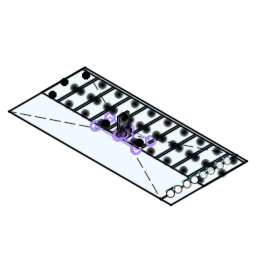
RIS-fusion360 (Autodesk Fusion 360 design; units mm, degrees)
Autodesk Fusion 360 part; units mm, degrees
sketch "Sketch1" plane through (0, 0, 0) normal (1, 0, 0) x (0, 1, 0)
  line L0 (9.4, 3.95) -> (-9.4, 3.95)
  line L1 (-9.4, 3.95) -> (-9.4, -3.95)
  line L2 (-9.4, -3.95) -> (9.4, -3.95)
  line L3 (9.4, -3.95) -> (9.4, 3.95)
  line L4 (9.4, 3.95) -> (-9.4, -3.95) construction
  line L5 (-9.4, 3.95) -> (9.4, -3.95) construction
  circle A0 centre (0, -0.1) radius 1.45
  line L6 (0, 3.95) -> (0, -3.95) construction
  line L7 (0, -3.95) -> (0, -7.55) construction
  line L8 (0, -7.55) -> (-2.05, -7.55)
  line L9 (0, -7.55) -> (2.05, -7.55)
  line L10 (-2.05, -7.55) -> (-2.05, -3.95)
  line L11 (2.05, -7.55) -> (2.05, -3.95)
  line L12 (0, -7.55) -> (-7.5, -7.55)
  line L13 (0, -7.55) -> (7.5, -7.55)
  line L14 (-7.5, -7.55) -> (-7.5, -10)
  line L15 (-7.5, -10) -> (7.5, -10)
  line L16 (7.5, -10) -> (7.5, -7.55)
  circle A1 centre (0, 3.3786) radius 5.7286
  point P0 (0, -3.95)
  point P1 (0, -2.35)
  point P2 (5.7, 3.95)
  point P3 (-5.7, 3.95)
  dimension "d1" = 18.8
  dimension "d2" = 7.9
  dimension "d3" = 2.9
  dimension "d4" = 4.05
  dimension "d7" = 3.6
  dimension "d8" = 2.05
  dimension "d9" = 2.05
  dimension "d10" = 7.5
  dimension "d11" = 7.5
  dimension "d12" = 2.45
  dimension "d19" = 6.3
  dimension "d20" = 5.7
  dimension "d21" = 5.7
  constraint horizontal L0
  constraint perpendicular L0 L1
  constraint parallel L0 L2
  constraint parallel L1 L3
  constraint coincident L4 origin
  constraint coincident L5 origin
  constraint midpoint L0 L6.start
  constraint coincident A0.centre L6
  constraint coincident P0 L6.end
  constraint midpoint L2 P0
  constraint perpendicular L2 L7
  constraint perpendicular L7 L8
  constraint perpendicular L7 L9
  constraint coincident L2 L10.end
  constraint perpendicular L2 L10
  constraint coincident L2 L11.end
  constraint perpendicular L2 L11
  constraint perpendicular L7 L12
  constraint perpendicular L7 L13
  constraint perpendicular L12 L14
  constraint perpendicular L14 L15
  constraint vertical L16
  constraint coincident L6 P1
  constraint coincident L0 P2
  constraint coincident L0 P3
  constraint coincident P2 A1
  constraint coincident P1 A1
  constraint coincident P3 A1
  measures "d1" distance of L0.start L0.end
  measures "d2" distance of L0.start L2.end
  measures "d3" diameter of A0
  measures "d4" distance of L0 A0.centre
  measures "d7" distance of P0 L7.end
  measures "d8" distance of L7.end L8.end
  measures "d9" distance of L7.end L9.end
  measures "d10" distance of L7.end L12.end
  measures "d11" distance of L7.end L13.end
  measures "d12" distance of L13.end L15.end
  measures "d19" distance of L0 P1
  measures "d20" distance of L6.start P2
  measures "d21" distance of L6.start P3
extrude "Extrude1" add sketch "Sketch1" along normal blind 4.5 contours A0 makes body 1
extrude "Extrude2" add sketch "Sketch1" against normal blind 2.5 separate body contours L0 L1 L2 L3 A1 | L2 L8 L9 L10 L11 L12 L13 makes body 2
extrude "Extrude4" add sketch "Sketch1" against normal blind 1.2 contours L0 A1 picked at (0.0361, 3.082) bodies 2 1
extrude "Extrude3" add sketch "Sketch1" against normal blind 7 contours L8 L9 L12 L13 L14 L15 L16 bodies 2
sketch "Sketch2" plane through (0, 0, 0) normal (1, 0, 0) x (0, 1, 0)
  circle A0 centre (0, -0.1) radius 1.45
  line L0 (-9.4, 3.95) -> (-9.4, -3.95)
  line L1 (-9.4, -3.95) -> (-2.05, -3.95)
  line L2 (-2.05, -3.95) -> (-2.05, -7.55)
  line L3 (-2.05, -7.55) -> (-7.5, -7.55)
  line L4 (-7.5, -7.55) -> (-7.5, -10)
  line L5 (-7.5, -10) -> (7.5, -10)
  line L6 (7.5, -10) -> (7.5, -7.55)
  line L7 (7.5, -7.55) -> (2.05, -7.55)
  line L8 (2.05, -7.55) -> (2.05, -3.95)
  line L9 (2.05, -3.95) -> (9.4, -3.95)
  line L10 (9.4, -3.95) -> (9.4, 3.95)
  line L11 (9.4, 3.95) -> (-9.4, 3.95)
  line L12 (-7.5, -8.775) -> (7.5, -8.775)
  circle A1 centre (0, -0.1) radius 1.65
  line L13 (9.6, -3.95) -> (9.6, 4.15)
  line L14 (9.6, 4.15) -> (-9.6, 4.15)
  line L15 (-9.6, 4.15) -> (-9.6, -3.95)
  line L16 (-2.05, -7.35) -> (-7.5, -7.35)
  line L17 (7.5, -7.35) -> (2.05, -7.35)
  line L18 (-9.6, -4.15) -> (-7.5, -7.35)
  line L19 (9.6, -4.15) -> (7.5, -7.35)
  line L20 (-9.4, -4.15) -> (-2.25, -4.15)
  line L21 (-2.25, -4.15) -> (-2.25, -7.55)
  line L22 (2.25, -7.55) -> (2.25, -4.15)
  line L23 (2.25, -4.15) -> (9.4, -4.15)
  line L24 (-9.4, -4.15) -> (-9.6, -4.15)
  line L25 (9.4, -4.15) -> (9.6, -4.15)
  line L26 (-2.05, -7.35) -> (2.05, -7.35)
  line L27 (-9.6, -3.95) -> (-19.4, -3.95)
  line L28 (-19.4, -3.95) -> (-19.4, 8.95)
  line L29 (-19.4, 8.95) -> (19.4, 8.95)
  line L30 (9.6, -3.95) -> (19.4, -3.95)
  line L31 (19.4, -3.95) -> (19.4, 8.95)
  line L32 (19.4, -3.95) -> (7.5, -7.35)
  line L33 (-19.4, -3.95) -> (-7.5, -7.35)
  line L34 (9.6, -3.95) -> (9.6, -4.15)
  line L35 (-9.6, -3.95) -> (-9.6, -4.15)
  circle A2 centre (-14.4, 1.85) radius 2.1
  line L36 (-9.4, 1.85) -> (-19.4, 1.85) construction
  line L37 (0, 3.95) -> (0, 8.95) construction
  circle A3 centre (14.4, 1.85) radius 2.1
  line L38 (-2.05, -3.95) -> (-9.4, -3.95)
  dimension "d29" = 0.2
  dimension "d45" = 0.2
  dimension "d46" = 0.2
  dimension "d47" = 0.2
  dimension "d48" = 0.2
  dimension "d49" = 0.2
  dimension "d60" = 5
  dimension "d63" = 10
  dimension "d68" = 4.2
  dimension "d99" = 5.8
  constraint midpoint L4 L12.start
  constraint midpoint L6 L12.end
  constraint parallel L20 L24
  constraint parallel L23 L25
  constraint perpendicular L8 L26
  constraint perpendicular L15 L27
  constraint perpendicular L27 L28
  constraint perpendicular L28 L29
  constraint perpendicular L13 L30
  constraint perpendicular L30 L31
  constraint equal L27 L30
  constraint perpendicular L30 L34
  constraint perpendicular L27 L35
  constraint coincident L28 L36.end
  constraint perpendicular L28 L36
  constraint midpoint A2.centre L36
  constraint midpoint L11 L37.start
  constraint midpoint L29 L37.end
  constraint symmetric A2 L37 A3
  constraint coincident L0 L36.start
  measures "d60" distance of L11 L29
  measures "d63" distance of L0 L28
  measures "d68" diameter of A2
  measures "d99" distance of L36 L38
extrude "Extrude5" add sketch "Sketch2" along normal blind 8 separate body contours L0 L1 L2 L8 L9 L10 L11 L26 L38 | L0 L1 L2 L8 L9 L10 L11 L13 L14 L15 L16 L17 L20 L21 L22 L23 L24 L25 L34 L35 L38 | L16 L18 L20 L21 L24 | L18 L27 L33 L35 | L17 L19 L22 L23 L25 | L13 L14 L15 L27 L28 L29 L30 L31 | L19 L30 L32 L34 makes body 3
sketch "Sketch3" plane through (-2.5, 0, 0) normal (-1, 0, 0) x (0, -1, 0)
  line L0 (9.4, -3.95) -> (9.4, 3.95)
  line L1 (9.4, 3.95) -> (5.7, 3.95)
  arc A0 (-5.7, 3.95) -> (5.7, 3.95) centre (0, 3.3786) ccw
  line L2 (-5.7, 3.95) -> (-9.4, 3.95)
  line L3 (-9.4, 3.95) -> (-9.4, -3.95)
  line L4 (-9.4, -3.95) -> (-2.05, -3.95)
  line L5 (-2.05, -3.95) -> (-2.05, -7.55)
  line L6 (-2.05, -7.55) -> (2.05, -7.55)
  line L7 (2.05, -7.55) -> (2.05, -3.95)
  line L8 (2.05, -3.95) -> (9.4, -3.95)
  arc A1 (-5.7, 3.95) -> (5.7, 3.95) centre (0, 3.3786) ccw
  line L9 (5.7, 3.95) -> (-5.7, 3.95)
  arc A2 (-5.501, 3.93) -> (5.501, 3.93) centre (0, 3.3786) ccw
  line L10 (-5.501, 3.93) -> (5.501, 3.93)
  line L11 (-2.05, -3.95) -> (2.05, -3.95)
  line L12 (-9.4, -3.95) -> (-2.05, -3.95) construction
  line L13 (-2.05, -3.95) -> (-2.05, -7.55) construction
  line L14 (2.05, -7.55) -> (2.05, -3.95) construction
  line L15 (2.05, -3.95) -> (9.4, -3.95) construction
  line L16 (-9.4, 3.95) -> (-9.4, -3.95) construction
  line L17 (9.4, -3.95) -> (9.4, 3.95) construction
  line L18 (7.5, -7.55) -> (2.05, -7.55)
  line L19 (2.05, -7.55) -> (-2.05, -7.55)
  line L20 (-2.05, -7.55) -> (-7.5, -7.55)
  line L21 (-7.55, -7.35) -> (-2.05, -7.35)
  line L22 (7.55, -7.35) -> (2.05, -7.35)
  line L23 (19.4, -3.95) -> (19.4, 8.95)
  line L24 (19.4, 8.95) -> (-19.4, 8.95)
  line L25 (-19.4, 8.95) -> (-19.4, -3.95)
  line L26 (-19.4, -3.95) -> (-7.55, -7.35)
  line L27 (19.4, -3.95) -> (7.55, -7.35)
  line L28 (-9.4, -3.95) -> (-19.4, -3.95) construction
  line L29 (9.4, -3.95) -> (19.4, -3.95) construction
  dimension "d34" = 0.2
  dimension "d35" = 0.2
  dimension "d56" = 5.5
  dimension "d57" = 10
  dimension "d58" = 5.5
  dimension "d62" = 5
  constraint parallel L9 L10
  constraint coincident L4.end L5.start
  constraint coincident L7.end L8.start
  constraint coincident L13 L21.end
  constraint perpendicular L13 L21
  constraint coincident L14 L22.end
  constraint perpendicular L14 L22
  constraint perpendicular L23 L24
  constraint coincident L3.end L4.start
  constraint perpendicular L25 L28
  constraint coincident L0.start L8.end
  constraint perpendicular L23 L29
  constraint horizontal L24
  constraint vertical L25
  constraint equal L28 L29
  measures "d34" distance of L20 L21
  measures "d35" distance of L18 L22
  measures "d56" distance of L21.start L21.end
  measures "d57" distance of L23.start L0.start
  measures "d58" distance of L22.start L22.end
  measures "d62" distance of L9 L24
extrude "Extrude6" add sketch "Sketch3" against normal up to surface (1.1 mm away) separate body contours A2 L10 makes body 4
extrude "Extrude7" add sketch "Sketch3" along normal blind 3 separate body contours L0 L1 A0 L2 L3 L4 L8 A1 L11 | L0 L1 L2 L3 L4 L5 L7 L8 L9 L21 L22 L23 L24 L25 L26 L27 | A0 A1 L9 | A2 L10 makes body 5
combine "Combine1" operation add target body 4 tool bodies 5
extrude "Extrude10" add sketch "Sketch2" against normal up to surface (2.3 mm away) contours L16 L18 L20 L21 L24 | L18 L27 L33 L35 | L17 L19 L22 L23 L25 | L13 L14 L15 L27 L28 L29 L30 L31 | L19 L30 L32 L34 | A2 | A3 bodies 3
extrude "Extrude15" cut 2 faces at (0, 13.5612, 2.607) (0, -13.9454, 2.4562) along direction (1, 0, 0) up to surface end surface through (-2.3, 0, 0) normal (-1, 0, 0) offset 0 on bodies 3 bodies 3
sketch "Sketch5" plane through (0, 0, 8.95) normal (0, 0, 1) x (-1, 0, 0)
  line L0 (2.3, 19.4) -> (-8, 19.4)
  line L1 (-8, 19.4) -> (-8, -19.4)
  line L2 (-8, -19.4) -> (2.3, -19.4)
  line L3 (2.3, -19.4) -> (2.3, 19.4)
  line L4 (-4.6, -19.4) -> (-4.6, 19.4)
  dimension "d94" = 3.4
  constraint coincident L2 L4.start
  constraint coincident L0 L4.end
  constraint perpendicular L0 L4
  measures "d94" distance of L1 L4
extrude "Extrude9" add sketch "Sketch5" along normal blind 58 separate body contours L0 L2 L3 L4 makes body 6
sketch "Sketch7" plane through (-5.5, 0, 0) normal (-1, 0, 0) x (0, -1, 0)
  line L0 (19.4, 8.95) -> (-19.4, 8.95)
  line L1 (-19.4, 8.95) -> (-19.4, -3.95)
  line L2 (-19.4, -3.95) -> (-7.55, -7.35)
  line L3 (-7.55, -7.35) -> (-2.05, -7.35)
  line L4 (-2.05, -7.35) -> (-2.05, -3.95)
  line L5 (-2.05, -3.95) -> (2.05, -3.95)
  line L6 (2.05, -3.95) -> (2.05, -7.35)
  line L7 (2.05, -7.35) -> (7.55, -7.35)
  line L8 (7.55, -7.35) -> (19.4, -3.95)
  line L9 (19.4, -3.95) -> (19.4, 8.95)
  circle A0 centre (14.4, 1.85) radius 2.1
  circle A1 centre (-14.4, 1.85) radius 2.1
extrude "Extrude11" cut sketch "Sketch7" against normal up to surface (3 mm away) contours A0 | A1 bodies 4
sketch "Sketch8" plane through (4.6, 0, 0) normal (1, 0, 0) x (0, 1, 0)
  line L0 (-19.4, 8.95) -> (19.4, 8.95)
  line L1 (19.4, 8.95) -> (19.4, 66.95)
  line L2 (19.4, 66.95) -> (-19.4, 66.95)
  line L3 (-19.4, 66.95) -> (-19.4, 8.95)
  line L4 (0, 66.95) -> (0, 8.95) construction
  circle A0 centre (-13, 23.95) radius 2.25
  circle A1 centre (13, 23.95) radius 2.25
  circle A2 centre (0, 58.95) radius 2.25
  line L5 (19.4, 8.95) -> (-19.4, 8.95)
  dimension "d95" = 4.5
  dimension "d100" = 13
  dimension "d101" = 15
  dimension "d102" = 4.5
  dimension "d103" = 50
  constraint midpoint L2 L4.start
  constraint midpoint L0 L4.end
  constraint symmetric L4 A0 A1
  constraint coincident L4 A2.centre
  measures "d95" diameter of A0
  measures "d100" distance of L4 A0.centre
  measures "d101" distance of L0 A0.centre
  measures "d102" diameter of A2
  measures "d103" distance of A2.centre L5
extrude "Extrude16" cut sketch "Sketch8" against normal up to surface (6.9 mm away) contours A0 | A1 | A2 bodies 6
combine "Combine4" operation add target body 3 tool bodies 6
sketch "Motor Mount" plane through (0, 0, 0) normal (0, 0, 1) x (1, 0, 0)
  line L0 (80, 29) -> (-80, 29)
  line L1 (-80, 29) -> (-80, -29)
  line L2 (-80, -29) -> (80, -29)
  line L3 (80, -29) -> (80, 29)
  circle A0 centre (0, -20) radius 2.15
  circle A1 centre (-67, 0) radius 2.15
  line L4 (-47, 0) -> (-47, -7.6)
  line L5 (-47, -7.6) -> (-36.1, -7.6)
  line L6 (-36.1, -7.6) -> (-36.1, -5.5)
  line L7 (-36.1, -5.5) -> (-28.1, -5.5)
  line L8 (-28.1, -5.5) -> (-28.1, -7.6)
  line L9 (-28.1, -7.6) -> (0, -7.6)
  line L10 (0, 0) -> (0, -29) construction
  line L11 (0, 0) -> (-80, 0) construction
  line L12 (0, 1.75) -> (0, 22.5) construction
  line L13 (47, 0) -> (47, -7.6)
  line L14 (47, -7.6) -> (36.1, -7.6)
  line L15 (36.1, -7.6) -> (36.1, -5.5)
  line L16 (36.1, -5.5) -> (28.1, -5.5)
  line L17 (28.1, -5.5) -> (28.1, -7.6)
  line L18 (28.1, -7.6) -> (0, -7.6)
  line L19 (1.75, 0) -> (22.5, 0) construction
  line L20 (-47, 0) -> (-47, 7.6)
  line L21 (-47, 7.6) -> (-36.1, 7.6)
  line L22 (-36.1, 7.6) -> (-36.1, 5.5)
  line L23 (-36.1, 5.5) -> (-28.1, 5.5)
  line L24 (-28.1, 5.5) -> (-28.1, 7.6)
  line L25 (-28.1, 7.6) -> (0, 7.6)
  line L26 (47, 0) -> (47, 7.6)
  line L27 (47, 7.6) -> (36.1, 7.6)
  line L28 (36.1, 7.6) -> (36.1, 5.5)
  line L29 (36.1, 5.5) -> (28.1, 5.5)
  line L30 (28.1, 5.5) -> (28.1, 7.6)
  line L31 (28.1, 7.6) -> (0, 7.6)
  circle A2 centre (65, 0) radius 2.15
  circle A3 centre (0, 20) radius 2.15
  line L32 (-28.35, 7.85) -> (0, 7.85)
  line L33 (28.35, 7.85) -> (0, 7.85)
  line L34 (28.35, 5.75) -> (28.35, 7.85)
  line L35 (35.85, 5.75) -> (28.35, 5.75)
  line L36 (35.85, 7.85) -> (35.85, 5.75)
  line L37 (47.25, 7.85) -> (35.85, 7.85)
  line L38 (47.25, 0) -> (47.25, 7.85)
  line L39 (47.25, 0) -> (47.25, -7.85)
  line L40 (47.25, -7.85) -> (35.85, -7.85)
  line L41 (35.85, -7.85) -> (35.85, -5.75)
  line L42 (35.85, -5.75) -> (28.35, -5.75)
  line L43 (28.35, -5.75) -> (28.35, -7.85)
  line L44 (28.35, -7.85) -> (0, -7.85)
  line L45 (-28.35, -7.85) -> (0, -7.85)
  line L46 (-28.35, -5.75) -> (-28.35, -7.85)
  line L47 (-35.85, -5.75) -> (-28.35, -5.75)
  line L48 (-35.85, -7.85) -> (-35.85, -5.75)
  line L49 (-47.25, -7.85) -> (-35.85, -7.85)
  line L50 (-47.25, 0) -> (-47.25, -7.85)
  line L51 (-47.25, 0) -> (-47.25, 7.85)
  line L52 (-47.25, 7.85) -> (-35.85, 7.85)
  line L53 (-35.85, 7.85) -> (-35.85, 5.75)
  line L54 (-35.85, 5.75) -> (-28.35, 5.75)
  line L55 (-28.35, 5.75) -> (-28.35, 7.85)
  line L56 (0, 0) -> (80, 0) construction
  line L57 (6.2897, -23.5719) -> (64.2897, -23.5719) construction
  line L58 (64.2897, -23.5719) -> (64.2897, -15.4585) construction
  line L59 (64.2897, -15.4585) -> (6.2897, -15.4585) construction
  line L60 (6.2897, -15.4585) -> (6.2897, -23.5719) construction
  line L61 (62.7995, -15.5811) -> (63.8445, -15.5811)
  spline S0 degree 3 poles (63.8445, -15.5811) (64.1057, -15.2618) (65.0347, -14.42) (66.2829, -14.42) knots 0 0 0 0 1 1 1 1
  line L62 (66.2829, -14.42) -> (66.3119, -14.42)
  spline S1 degree 3 poles (66.3119, -14.42) (67.2118, -14.42) (67.8504, -14.5071) (68.46, -15.2908) knots 0 0 0 0 1 1 1 1
  line L63 (68.46, -15.2908) -> (76.588, -15.2908)
  spline S2 degree 3 poles (76.588, -15.2908) (77.3137, -15.2908) (77.8943, -15.8714) (77.8943, -16.5971) knots 0 0 0 0 1 1 1 1
  spline S3 degree 3 poles (77.8943, -16.5971) (77.8943, -17.3228) (77.3137, -17.9034) (76.588, -17.9034) knots 0 0 0 0 1 1 1 1
  line L64 (76.588, -17.9034) -> (73.5981, -17.8453)
  spline S4 degree 3 poles (73.5981, -17.8453) (73.7432, -18.0485) (73.8303, -18.3098) (73.8303, -18.571) knots 0 0 0 0 1 1 1 1
  spline S5 degree 3 poles (73.8303, -18.571) (73.8303, -19.2387) (73.3659, -19.7612) (72.7563, -19.8773) knots 0 0 0 0 1 1 1 1
  spline S6 degree 3 poles (72.7563, -19.8773) (72.7853, -19.9354) (72.8143, -19.9644) (72.8433, -20.0225) knots 0 0 0 0 1 1 1 1
  spline S7 degree 3 poles (72.8433, -20.0225) (72.9885, -20.3418) (73.0175, -20.6901) (72.9014, -21.0094) knots 0 0 0 0 1 1 1 1
  line L65 (72.9014, -21.0094) -> (72.8724, -21.0675)
  spline S8 degree 3 poles (72.8724, -21.0675) (72.8377, -21.1718) (72.79, -21.2689) (72.7321, -21.3579) knots 0 0 0 0 1 1 1 1
  spline S9 degree 3 poles (72.7321, -21.3579) (72.614, -21.5573) (72.4315, -21.7192) (72.2047, -21.8222) knots 0 0 0 0 1 1 1 1
  spline S10 degree 3 poles (72.2047, -21.8222) (72.0425, -21.9033) (71.8801, -21.9586) (71.6944, -21.9659) knots 0 0 0 0 1 1 1 1
  spline S11 degree 3 poles (71.6944, -21.9659) (71.775, -22.2169) (71.7761, -22.4985) (71.6822, -22.7802) knots 0 0 0 0 1 1 1 1
  spline S12 degree 3 poles (71.6822, -22.7802) (71.5661, -23.1285) (71.3339, -23.3898) (71.0145, -23.5349) knots 0 0 0 0 1 1 1 1
  spline S13 degree 3 poles (71.0145, -23.5349) (70.997, -23.5424) (70.9799, -23.5494) (70.9628, -23.5565) knots 0 0 0 0 1 1 1 1
  spline S14 degree 3 poles (70.9628, -23.5565) (70.9343, -23.5688) (70.9055, -23.5803) (70.8762, -23.5906) knots 0 0 0 0 1 1 1 1
  spline S15 degree 3 poles (70.8762, -23.5906) (70.7284, -23.6457) (70.5897, -23.68) (70.4339, -23.68) knots 0 0 0 0 1 1 1 1
  spline S16 degree 3 poles (70.4339, -23.68) (70.3222, -23.68) (70.2106, -23.6626) (70.1121, -23.6282) knots 0 0 0 0 1 1 1 1
  spline S17 degree 3 poles (70.1121, -23.6282) (70.1033, -23.6261) (70.0944, -23.6243) (70.0856, -23.622) knots 0 0 0 0 1 1 1 1
  spline S18 degree 3 poles (70.0856, -23.622) (69.7663, -23.7091) (68.518, -23.9994) (67.444, -23.9994) knots 0 0 0 0 1 1 1 1
  spline S19 degree 3 poles (67.444, -23.9994) (65.412, -23.9994) (65.0056, -23.9703) (63.8735, -23.1285) knots 0 0 0 0 1 1 1 1
  line L66 (63.8735, -23.1285) -> (62.7994, -23.1285)
  spline S20 degree 3 poles (62.7994, -23.1285) (62.1317, -23.1285) (61.6383, -22.635) (61.6383, -21.9964) knots 0 0 0 0 1 1 1 1
  line L67 (61.6383, -21.9964) -> (61.6383, -16.7423)
  spline S21 degree 3 poles (61.6383, -16.7423) (61.6383, -16.1036) (62.1608, -15.5811) (62.7995, -15.5811) knots 0 0 0 0 1 1 1 1
  spline S22 degree 3 poles (76.588, -17.3228) (76.9944, -17.3228) (77.3137, -17.0035) (77.3137, -16.5971) knots 0 0 0 0 1 1 1 1
  spline S23 degree 3 poles (77.3137, -16.5971) (77.3137, -16.1907) (76.9944, -15.8714) (76.588, -15.8714) knots 0 0 0 0 1 1 1 1
  line L68 (76.588, -15.8714) -> (68.8955, -15.8714)
  spline S24 degree 3 poles (68.8955, -15.8714) (68.9041, -15.88) (68.9099, -15.8886) (68.9142, -15.8972) knots 0 0 0 0 1 1 1 1
  spline S25 degree 3 poles (68.9142, -15.8972) (69.2775, -16.3833) (69.663, -16.9017) (69.9793, -17.3315) knots 0 0 0 0 1 1 1 1
  spline S26 degree 3 poles (69.9793, -17.3315) (70.0036, -17.326) (70.0293, -17.3228) (70.0566, -17.3228) knots 0 0 0 0 1 1 1 1
  line L69 (70.0566, -17.3228) -> (72.524, -17.3228)
  spline S27 degree 3 poles (72.524, -17.3228) (72.5531, -17.3228) (72.5531, -17.3228) (72.5821, -17.3228) knots 0 0 0 0 1 1 1 1
  line L70 (72.5821, -17.3228) -> (76.588, -17.3228)
  spline S28 degree 3 poles (73.2207, -18.6291) (73.2207, -18.4259) (73.1627, -18.2517) (73.0175, -18.1066) knots 0 0 0 0 1 1 1 1
  spline S29 degree 3 poles (73.0175, -18.1066) (72.9014, -17.9905) (72.7272, -17.9034) (72.5531, -17.9034) knots 0 0 0 0 1 1 1 1
  line L71 (72.5531, -17.9034) -> (70.3967, -17.9034)
  spline S30 degree 3 poles (70.3967, -17.9034) (70.4435, -17.9685) (70.4855, -18.0271) (70.5211, -18.0776) knots 0 0 0 0 1 1 1 1
  spline S31 degree 3 poles (70.5211, -18.0776) (70.7612, -18.4378) (70.87, -18.7447) (70.903, -18.9982) knots 0 0 0 0 1 1 1 1
  spline S32 degree 3 poles (70.903, -18.9982) (70.9111, -19.0006) (70.9193, -19.0032) (70.9275, -19.0065) knots 0 0 0 0 1 1 1 1
  line L72 (70.9275, -19.0065) -> (71.7839, -19.3063)
  line L73 (71.7839, -19.3063) -> (72.3789, -19.3839)
  line L74 (72.3789, -19.3839) -> (72.495, -19.3839)
  spline S33 degree 3 poles (72.495, -19.3839) (72.9014, -19.3839) (73.2207, -19.0355) (73.2207, -18.6291) knots 0 0 0 0 1 1 1 1
  spline S34 degree 3 poles (70.1727, -23.0415) (70.3469, -23.0995) (70.5501, -23.0995) (70.7243, -23.0124) knots 0 0 0 0 1 1 1 1
  spline S35 degree 3 poles (70.7243, -23.0124) (70.7689, -22.9901) (70.8117, -22.9639) (70.8515, -22.9344) knots 0 0 0 0 1 1 1 1
  spline S36 degree 3 poles (70.8515, -22.9344) (70.9392, -22.8548) (71.0071, -22.7535) (71.0436, -22.6351) knots 0 0 0 0 1 1 1 1
  spline S37 degree 3 poles (71.0436, -22.6351) (71.1016, -22.4609) (71.1016, -22.2577) (71.0145, -22.0836) knots 0 0 0 0 1 1 1 1
  spline S38 degree 3 poles (71.0145, -22.0836) (70.9275, -21.9094) (70.7823, -21.7643) (70.6081, -21.7062) knots 0 0 0 0 1 1 1 1
  spline S39 degree 3 poles (70.6081, -21.7062) (70.5664, -21.6895) (70.5298, -21.663) (70.4997, -21.6306) knots 0 0 0 0 1 1 1 1
  line L75 (70.4997, -21.6306) -> (67.8795, -20.7192)
  spline S40 degree 3 poles (67.8795, -20.7192) (67.8396, -20.7053) (67.8009, -20.6896) (67.7634, -20.6723) knots 0 0 0 0 1 1 1 1
  line L76 (67.7634, -20.6723) -> (67.6472, -20.6321)
  spline S41 degree 3 poles (67.6472, -20.6321) (67.5601, -20.6031) (67.5021, -20.6031) (67.415, -20.6031) knots 0 0 0 0 1 1 1 1
  spline S42 degree 3 poles (67.415, -20.6031) (67.2989, -20.6031) (67.2118, -20.6321) (67.0957, -20.6612) knots 0 0 0 0 1 1 1 1
  spline S43 degree 3 poles (67.0957, -20.6612) (66.9215, -20.7483) (66.7764, -20.8934) (66.7183, -21.0676) knots 0 0 0 0 1 1 1 1
  spline S44 degree 3 poles (66.7183, -21.0676) (66.6602, -21.2418) (66.6602, -21.445) (66.7473, -21.6191) knots 0 0 0 0 1 1 1 1
  spline S45 degree 3 poles (66.7473, -21.6191) (66.8344, -21.7933) (66.9795, -21.9384) (67.1537, -21.9965) knots 0 0 0 0 1 1 1 1
  line L77 (67.1537, -21.9965) -> (70.1727, -23.0415)
  spline S46 degree 3 poles (69.7953, -20.2257) (69.7815, -20.2257) (69.7672, -20.2252) (69.7528, -20.2246) knots 0 0 0 0 1 1 1 1
  spline S47 degree 3 poles (69.7528, -20.2246) (69.596, -20.2247) (69.4424, -20.1977) (69.3019, -20.1386) knots 0 0 0 0 1 1 1 1
  spline S48 degree 3 poles (69.3019, -20.1386) (68.9245, -19.9935) (68.3729, -19.6161) (67.7343, -19.1226) knots 0 0 0 0 1 1 1 1
  spline S49 degree 3 poles (67.7343, -19.1226) (67.7053, -19.1516) (67.7053, -19.1807) (67.6763, -19.2387) knots 0 0 0 0 1 1 1 1
  line L78 (67.6763, -19.2387) -> (67.6472, -19.2968)
  spline S50 degree 3 poles (67.6472, -19.2968) (67.5552, -19.5958) (67.6461, -19.9126) (67.8753, -20.0892) knots 0 0 0 0 1 1 1 1
  line L79 (67.8753, -20.0892) -> (70.8694, -21.1256)
  spline S51 degree 3 poles (70.8694, -21.1256) (70.9741, -21.1605) (71.0708, -21.2087) (71.159, -21.2667) knots 0 0 0 0 1 1 1 1
  line L80 (71.159, -21.2667) -> (71.4209, -21.3578)
  spline S52 degree 3 poles (71.4209, -21.3578) (71.4619, -21.3715) (71.5029, -21.3817) (71.5438, -21.3886) knots 0 0 0 0 1 1 1 1
  spline S53 degree 3 poles (71.5438, -21.3886) (71.7669, -21.4122) (71.9848, -21.3392) (72.1336, -21.1878) knots 0 0 0 0 1 1 1 1
  spline S54 degree 3 poles (72.1336, -21.1878) (72.2053, -21.1124) (72.2584, -21.0224) (72.2918, -20.9223) knots 0 0 0 0 1 1 1 1
  line L81 (72.2918, -20.9223) -> (72.3208, -20.8643)
  spline S55 degree 3 poles (72.3208, -20.8643) (72.3638, -20.7246) (72.3668, -20.5811) (72.3346, -20.4497) knots 0 0 0 0 1 1 1 1
  spline S56 degree 3 poles (72.3346, -20.4497) (72.3238, -20.4137) (72.3098, -20.3777) (72.2918, -20.3417) knots 0 0 0 0 1 1 1 1
  spline S57 degree 3 poles (72.2918, -20.3417) (72.2047, -20.1676) (72.0595, -20.0514) (71.8854, -19.9934) knots 0 0 0 0 1 1 1 1
  line L82 (71.8854, -19.9934) -> (71.566, -19.8773)
  spline S58 degree 3 poles (71.566, -19.8773) (71.5425, -19.8655) (71.5203, -19.8501) (71.4999, -19.8319) knots 0 0 0 0 1 1 1 1
  line L83 (71.4999, -19.8319) -> (70.9564, -19.645)
  spline S59 degree 3 poles (70.9564, -19.645) (70.8012, -19.852) (70.5653, -20.0184) (70.3026, -20.119) knots 0 0 0 0 1 1 1 1
  spline S60 degree 3 poles (70.3026, -20.119) (70.1458, -20.1889) (69.9706, -20.2257) (69.7953, -20.2257) knots 0 0 0 0 1 1 1 1
  spline S61 degree 3 poles (62.2189, -21.9964) (62.2189, -22.2867) (62.4802, -22.5479) (62.7995, -22.5479) knots 0 0 0 0 1 1 1 1
  line L84 (62.7995, -22.5479) -> (63.9316, -22.5479)
  spline S62 degree 3 poles (63.9316, -22.5479) (64.0187, -22.5479) (64.1058, -22.5479) (64.1638, -22.606) knots 0 0 0 0 1 1 1 1
  spline S63 degree 3 poles (64.1638, -22.606) (65.2088, -23.3898) (65.4411, -23.4188) (67.4731, -23.4188) knots 0 0 0 0 1 1 1 1
  spline S64 degree 3 poles (67.4731, -23.4188) (67.9919, -23.4188) (68.5715, -23.3396) (69.0474, -23.2537) knots 0 0 0 0 1 1 1 1
  line L85 (69.0474, -23.2537) -> (67.0086, -22.548)
  spline S65 degree 3 poles (67.0086, -22.548) (66.6603, -22.4319) (66.399, -22.1996) (66.2539, -21.8803) knots 0 0 0 0 1 1 1 1
  spline S66 degree 3 poles (66.2539, -21.8803) (66.1088, -21.59) (66.0797, -21.2126) (66.1958, -20.8933) knots 0 0 0 0 1 1 1 1
  spline S67 degree 3 poles (66.1958, -20.8933) (66.3119, -20.545) (66.5441, -20.2837) (66.8635, -20.1386) knots 0 0 0 0 1 1 1 1
  spline S68 degree 3 poles (66.8635, -20.1386) (66.9486, -20.0961) (67.0412, -20.0638) (67.1376, -20.042) knots 0 0 0 0 1 1 1 1
  spline S69 degree 3 poles (67.1376, -20.042) (67.0073, -19.7539) (66.9832, -19.417) (67.0957, -19.0936) knots 0 0 0 0 1 1 1 1
  line L86 (67.0957, -19.0936) -> (67.1247, -19.0355)
  spline S70 degree 3 poles (67.1247, -19.0355) (67.1696, -18.9309) (67.23, -18.8265) (67.3016, -18.7298) knots 0 0 0 0 1 1 1 1
  spline S71 degree 3 poles (67.3016, -18.7298) (66.5343, -18.0629) (65.8519, -17.3332) (65.6733, -16.9165) knots 0 0 0 0 1 1 1 1
  spline S72 degree 3 poles (65.6733, -16.9165) (65.6152, -16.7713) (65.6733, -16.5971) (65.8184, -16.5391) knots 0 0 0 0 1 1 1 1
  spline S73 degree 3 poles (65.8184, -16.5391) (65.9635, -16.481) (66.1377, -16.5391) (66.1958, -16.6842) knots 0 0 0 0 1 1 1 1
  spline S74 degree 3 poles (66.1958, -16.6842) (66.34, -17.0368) (67.0505, -17.7786) (67.8192, -18.4359) knots 0 0 0 0 1 1 1 1
  spline S75 degree 3 poles (67.8192, -18.4359) (67.8501, -18.4468) (67.8802, -18.4627) (67.9085, -18.484) knots 0 0 0 0 1 1 1 1
  spline S76 degree 3 poles (67.9085, -18.484) (68.5471, -19.0355) (69.1567, -19.4419) (69.5341, -19.5871) knots 0 0 0 0 1 1 1 1
  spline S77 degree 3 poles (69.5341, -19.5871) (69.7327, -19.6593) (70.0325, -19.5967) (70.2656, -19.4622) knots 0 0 0 0 1 1 1 1
  spline S78 degree 3 poles (70.2656, -19.4622) (70.4321, -19.2293) (70.372, -18.8557) (70.0566, -18.3969) knots 0 0 0 0 1 1 1 1
  spline S79 degree 3 poles (70.0566, -18.3969) (69.7083, -17.9034) (68.7793, -16.6552) (68.0827, -15.7553) knots 0 0 0 0 1 1 1 1
  spline S80 degree 2 poles (68.0827, -15.7553) (68.0827, -15.7553) (68.0826, -15.7553) knots 0 0 0 1 1 1
  spline S81 degree 3 poles (68.0826, -15.7553) (67.5891, -15.0586) (67.1827, -15.0005) (66.2829, -15.0005) knots 0 0 0 0 1 1 1 1
  line L87 (66.2829, -15.0005) -> (66.2539, -15.0005)
  spline S82 degree 2 poles (66.2539, -15.0005) (65.0637, -15.0005) (64.1928, -16.0455) knots 0 0 0 1 1 1
  spline S83 degree 3 poles (64.1928, -16.0455) (64.1348, -16.1326) (64.0477, -16.1617) (63.9606, -16.1617) knots 0 0 0 0 1 1 1 1
  line L88 (63.9606, -16.1617) -> (62.7995, -16.1617)
  spline S84 degree 3 poles (62.7995, -16.1617) (62.4802, -16.1617) (62.2189, -16.4229) (62.2189, -16.7422) knots 0 0 0 0 1 1 1 1
  line L89 (62.2189, -16.7422) -> (62.2189, -21.9964)
  point P0 (0, 5.5)
  dimension "d111" = 58
  dimension "d112" = 160
  dimension "d114" = 4.3
  dimension "d117" = 8
  dimension "d118" = 47
  dimension "d119" = 2.1
  dimension "d120" = 7.6
  dimension "d121" = 28.1
  dimension "d122" = 13
  dimension "d123" = 4.3
  dimension "d124" = 9
  dimension "d125" = -0.25
  dimension "d126" = 15
  dimension "d127" = 4.3
  dimension "d129" = 7.5
  constraint horizontal L0
  constraint perpendicular L0 L1
  constraint parallel L0 L2
  constraint parallel L1 L3
  constraint perpendicular L4 L5
  constraint perpendicular L5 L6
  constraint perpendicular L6 L7
  constraint perpendicular L7 L8
  constraint perpendicular L8 L9
  constraint collinear L5 L9
  constraint vertical L4
  constraint coincident L10.start L11.start
  constraint midpoint L2 L10.end
  constraint perpendicular L2 L10
  constraint coincident L9.end L10
  constraint midpoint L1 L11.end
  constraint perpendicular L1 L11
  constraint coincident L4.start L11
  constraint coincident A1.centre L11
  constraint coincident A0.centre L10
  constraint symmetric L4.start L12 L13.start
  constraint symmetric L4.end L12 L13.end
  constraint symmetric L5.end L12 L14.end
  constraint symmetric L6.end L12 L15.end
  constraint symmetric L7.end L12 L16.end
  constraint symmetric L8.end L12 L17.end
  constraint symmetric L9.end L12 L18.end
  constraint symmetric L4.start L19 L20.start
  constraint symmetric L4.end L19 L20.end
  constraint symmetric L5.end L19 L21.end
  constraint symmetric L6.end L19 L22.end
  constraint symmetric L7.end L19 L23.end
  constraint symmetric L8.end L19 L24.end
  constraint symmetric L9.end L19 L25.end
  constraint symmetric L13.start L19 L26.start
  constraint symmetric L13.end L19 L26.end
  constraint symmetric L14.end L19 L27.end
  constraint symmetric L15.end L19 L28.end
  constraint symmetric L16.end L19 L29.end
  constraint symmetric L17.end L19 L30.end
  constraint symmetric A0 L19 A3
  constraint midpoint L3 L56.end
  constraint coincident A2.centre L56
  constraint horizontal L57
  measures "d111" distance of L0.start L2.end
  measures "d112" distance of L0.start L0.end
  measures "d114" diameter of A1
  measures "d117" distance of L6.end L7.end
  measures "d118" distance of L4 L9.end
  measures "d119" distance of L5 L7
  measures "d120" distance of L4.start L4.end
  measures "d121" distance of L8 L9.end
  measures "d122" distance of L1 A1.centre
  measures "d123" diameter of A0
  measures "d124" distance of L2 A0.centre
  measures "d126" distance of L3 A2.centre
  measures "d127" diameter of A2
sketch "Baae board" plane through (0, 0, 0) normal (0, 0, 1) x (1, 0, 0)
sketch "Base" plane through (0, 0, 0) normal (0, 0, 1) x (1, 0, 0)
  line L0 (300, 150) -> (-300, 150)
  line L1 (-300, 150) -> (-300, -150)
  line L2 (-300, -150) -> (300, -150)
  line L3 (300, -150) -> (300, 150)
  line L4 (300, 150) -> (-300, -150) construction
  line L5 (-300, 150) -> (300, -150) construction
  line L6 (-300, 140) -> (-242, 140)
  line L7 (-242, 140) -> (-242, -20)
  line L8 (-242, -20) -> (-300, -20)
  line L9 (-300, -20) -> (-300, 140)
  line L10 (-80, -29) -> (80, -29)
  line L11 (80, -29) -> (80, 29)
  line L12 (-80, 29) -> (-80, -29)
  line L13 (80, 29) -> (-80, 29)
  circle A0 centre (-67, 0) radius 2.15
  circle A1 centre (0, -20) radius 2.15
  circle A2 centre (0, 20) radius 2.15
  circle A3 centre (65, 0) radius 2.15
  circle A4 centre (-271, 125) radius 2.15
  circle A5 centre (-271, -7) radius 2.15
  line L14 (-80, 0) -> (-67, 0) construction
  line L15 (-271, 140) -> (-271, 125) construction
  line L16 (-271, -20) -> (-271, -7) construction
  line L17 (65, 0) -> (80, 0) construction
  line L18 (-300, 60) -> (-291, 60) construction
  circle A6 centre (-291, 60) radius 2.15
  line L19 (0, 29) -> (0, 20) construction
  circle A7 centre (-251, 60) radius 2.15
  line L20 (-177.3333, -20) -> (-235.3333, -20)
  line L21 (-235.3333, -20) -> (-235.3333, 140)
  line L22 (-235.3333, 140) -> (-177.3333, 140)
  line L23 (-177.3333, 140) -> (-177.3333, -20)
  circle A8 centre (-226.3333, 60) radius 2.15
  circle A9 centre (-186.3333, 60) radius 2.15
  circle A10 centre (-206.3333, 125) radius 2.15
  circle A11 centre (-206.3333, -7) radius 2.15
  line L24 (-112.6667, -20) -> (-170.6667, -20)
  line L25 (-170.6667, -20) -> (-170.6667, 140)
  line L26 (-170.6667, 140) -> (-112.6667, 140)
  line L27 (-112.6667, 140) -> (-112.6667, -20)
  circle A12 centre (-161.6667, 60) radius 2.15
  circle A13 centre (-121.6667, 60) radius 2.15
  circle A14 centre (-141.6667, 125) radius 2.15
  circle A15 centre (-141.6667, -7) radius 2.15
  line L28 (-48, -20) -> (-106, -20)
  line L29 (-106, -20) -> (-106, 140)
  line L30 (-106, 140) -> (-48, 140)
  line L31 (-48, 140) -> (-48, -20)
  circle A16 centre (-97, 60) radius 2.15
  circle A17 centre (-57, 60) radius 2.15
  circle A18 centre (-77, 125) radius 2.15
  circle A19 centre (-77, -7) radius 2.15
  line L32 (16.6667, -20) -> (-41.3333, -20)
  line L33 (-41.3333, -20) -> (-41.3333, 140)
  line L34 (-41.3333, 140) -> (16.6667, 140)
  line L35 (16.6667, 140) -> (16.6667, -20)
  circle A20 centre (-32.3333, 60) radius 2.15
  circle A21 centre (7.6667, 60) radius 2.15
  circle A22 centre (-12.3333, 125) radius 2.15
  circle A23 centre (-12.3333, -7) radius 2.15
  line L36 (81.3333, -20) -> (23.3333, -20)
  line L37 (23.3333, -20) -> (23.3333, 140)
  line L38 (23.3333, 140) -> (81.3333, 140)
  line L39 (81.3333, 140) -> (81.3333, -20)
  circle A24 centre (32.3333, 60) radius 2.15
  circle A25 centre (72.3333, 60) radius 2.15
  circle A26 centre (52.3333, 125) radius 2.15
  circle A27 centre (52.3333, -7) radius 2.15
  line L40 (146, -20) -> (88, -20)
  line L41 (88, -20) -> (88, 140)
  line L42 (88, 140) -> (146, 140)
  line L43 (146, 140) -> (146, -20)
  circle A28 centre (97, 60) radius 2.15
  circle A29 centre (137, 60) radius 2.15
  circle A30 centre (117, 125) radius 2.15
  circle A31 centre (117, -7) radius 2.15
  line L44 (210.6667, -20) -> (152.6667, -20)
  line L45 (152.6667, -20) -> (152.6667, 140)
  line L46 (152.6667, 140) -> (210.6667, 140)
  line L47 (210.6667, 140) -> (210.6667, -20)
  circle A32 centre (161.6667, 60) radius 2.15
  circle A33 centre (201.6667, 60) radius 2.15
  circle A34 centre (181.6667, 125) radius 2.15
  circle A35 centre (181.6667, -7) radius 2.15
  line L48 (275.3333, -20) -> (217.3333, -20)
  line L49 (217.3333, -20) -> (217.3333, 140)
  line L50 (217.3333, 140) -> (275.3333, 140)
  line L51 (275.3333, 140) -> (275.3333, -20)
  circle A36 centre (226.3333, 60) radius 2.15
  circle A37 centre (266.3333, 60) radius 2.15
  circle A38 centre (246.3333, 125) radius 2.15
  circle A39 centre (246.3333, -7) radius 2.15
  line L52 (340, -20) -> (282, -20)
  line L53 (282, -20) -> (282, 140)
  line L54 (282, 140) -> (340, 140)
  line L55 (340, 140) -> (340, -20)
  circle A40 centre (291, 60) radius 2.15
  circle A41 centre (331, 60) radius 2.15
  circle A42 centre (311, 125) radius 2.15
  circle A43 centre (311, -7) radius 2.15
  line L56 (300, 150) -> (340, 150)
  line L57 (340, 150) -> (340, -150)
  line L58 (340, -150) -> (300, -150)
  line L59 (300, -150) -> (300, 150)
  line L60 (300, 82.1191) -> (285, 82.1191)
  line L61 (285, 82.1191) -> (285, 112.1191)
  line L62 (285, 112.1191) -> (300, 112.1191)
  line L63 (300, 112.1191) -> (300, 82.1191)
  line L64 (300, 46.955) -> (285, 46.955)
  line L65 (285, 46.955) -> (285, 16.955)
  line L66 (285, 16.955) -> (300, 16.955)
  line L67 (300, 16.955) -> (300, 46.955)
  line L68 (1.75, 0) -> (22.5, 0)
  line L69 (285, -82.1191) -> (285, -112.1191)
  line L70 (300, -82.1191) -> (285, -82.1191)
  line L71 (285, -112.1191) -> (300, -112.1191)
  line L72 (300, -46.955) -> (285, -46.955)
  line L73 (285, -46.955) -> (285, -16.955)
  line L74 (285, -16.955) -> (300, -16.955)
  line L75 (300, 82.3191) -> (285.2, 82.3191)
  line L76 (285.2, 82.3191) -> (285.2, 111.9191)
  line L77 (285.2, 111.9191) -> (300, 111.9191)
  line L78 (300, 46.755) -> (285.2, 46.755)
  line L79 (285.2, 46.755) -> (285.2, 17.155)
  line L80 (285.2, 17.155) -> (300, 17.155)
  line L81 (300, -46.755) -> (285.2, -46.755)
  line L82 (285.2, -46.755) -> (285.2, -17.155)
  line L83 (285.2, -17.155) -> (300, -17.155)
  line L84 (300, -82.3191) -> (285.2, -82.3191)
  line L85 (285.2, -82.3191) -> (285.2, -111.9191)
  line L86 (285.2, -111.9191) -> (300, -111.9191)
  dimension "d130" = 600
  dimension "d131" = 300
  dimension "d132" = 4.3
  dimension "d133" = 4.3
  dimension "d134" = 4.3
  dimension "d135" = 0
  dimension "d136" = 10
  dimension "d140" = 582
  dimension "d141" = 10
  dimension "d143" = 55
  dimension "d144" = 15
  dimension "d145" = 30
  dimension "d147" = 0.2
  dimension "d149" = 0.2
  constraint horizontal L0
  constraint perpendicular L0 L1
  constraint parallel L0 L2
  constraint parallel L1 L3
  constraint coincident L4 origin
  constraint coincident L5 origin
  constraint horizontal L6
  constraint vertical L7
  constraint horizontal L8
  constraint vertical L9
  constraint equal L7 L13
  constraint equal L6 L12
  constraint coincident A0.centre L14.end
  constraint horizontal L14
  constraint midpoint L6 L15.start
  constraint coincident A4.centre L15.end
  constraint perpendicular L6 L15
  constraint midpoint L8 L16.start
  constraint coincident A5.centre L16.end
  constraint perpendicular L8 L16
  constraint equal L14 L16
  constraint coincident A3.centre L17.start
  constraint midpoint L11 L17.end
  constraint equal L15 L17
  constraint midpoint L12 L14.start
  constraint midpoint L9 L18.start
  constraint perpendicular L7 L18
  constraint coincident L18.end A6.centre
  constraint midpoint L13 L19.start
  constraint coincident A2.centre L19.end
  constraint equal L18 L19
  constraint symmetric L15 A6 A7
  constraint horizontal L56
  constraint vertical L57
  constraint horizontal L58
  constraint vertical L59
  constraint collinear L2 L58
  constraint horizontal L60
  constraint vertical L61
  constraint horizontal L62
  constraint vertical L63
  constraint coincident L3 L60.start
  constraint horizontal L64
  constraint vertical L65
  constraint horizontal L66
  constraint vertical L67
  constraint coincident L3 L64.start
  constraint equal L62 L64
  constraint equal L61 L65
  constraint symmetric L60.start L68 L70.start
  constraint symmetric L60.end L68 L69.start
  constraint symmetric L61.end L68 L69.end
  constraint symmetric L62.end L68 L71.end
  constraint symmetric L64.start L68 L72.start
  constraint symmetric L64.end L68 L72.end
  constraint symmetric L65.end L68 L73.end
  constraint symmetric L66.end L68 L74.end
  measures "d130" distance of L1.end L2.end
  measures "d131" distance of L0.end L1.end
  measures "d132" diameter of A4
  measures "d133" diameter of A5
  measures "d134" diameter of A6
  measures "d135" distance of L1 L9
  measures "d136" distance of L0 L6
  measures "d143" distance of L57 L61
  measures "d144" distance of L3 L61
  measures "d145" distance of L60.end L61.end
equation "d8 = ( 4.1 / 2 ) * 1 mm"
equation "d9 = ( 4.1 / 2 ) * 1 mm"
equation "d10 = ( 15 / 2 ) * 1 mm"
equation "d11 = ( 15 / 2 ) * 1 mm"
equation "d20 = ( 11.4 / 2 ) * 1 mm"
equation "d21 = ( 11.4 / 2 ) * 1 mm"
equation "d27 = -tol"
equation "tol = 0.2 mm"
equation "d29 = tol"
equation "d30 = tol"
equation "d34 = tol"
equation "d35 = tol"
equation "reflector_wall_wid = 4 mm"
equation "d45 = tol"
equation "d46 = tol"
equation "d47 = tol"
equation "d48 = tol"
equation "d49 = tol"
equation "d50 = tol"
equation "d57 = side_padding"
equation "side_padding = 10 mm"
equation "d60 = mount_rise"
equation "mount_rise = 5 mm"
equation "d62 = mount_rise"
equation "d63 = side_padding"
equation "d68 = screw_hole"
equation "screw_hole = 4.2 mm"
equation "d114 = screw_hole_laser"
equation "d118 = ( 94 / 2 ) * 1 mm"
equation "d121 = ( 56.2 / 2 ) * 1 mm"
equation "d123 = screw_hole_laser"
equation "d127 = screw_hole_laser"
equation "screw_hole_laser = 4.3 mm"
equation "d132 = screw_hole_laser"
equation "d133 = screw_hole_laser"
equation "d134 = screw_hole_laser"
equation "d135 = base_padding_x"
equation "base_padding_x = 0 mm"
equation "d140 = 600 mm + 55 mm - seam_wid - 2 * base_padding_x - 58 mm"
equation "d144 = seam_wid"
equation "seam_wid = 15 mm"
equation "d147 = tol"
equation "d148 = -tol"
equation "d149 = tol"
equation "d150 = -tol"
named bodies: "Motor Mount", "Adapter", "Lid"
